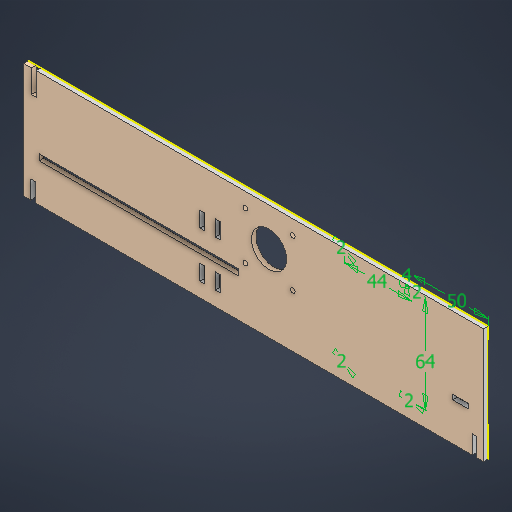
# Autodesk Inventor part: Sideboard
Saved by Autodesk Inventor 2027 (Build 310192000, 192)
## iProperties
Created: 2026-05-09
Part Number: Sideboard
Material: Generic
Document SubType Name: Modeling
Designer: alexy
Density: 1 g/cm^3
Appearance: Default
Author: alexy
Autodesk Inventor part; units mm, degrees
ref_plane "YZ Plane" through (0, 0, 0) normal (1, 0, 0) x (0, 1, 0)
ref_plane "XZ Plane" through (0, 0, 0) normal (0, 1, 0) x (-1, 0, 0)
ref_plane "XY Plane" through (0, 0, 0) normal (0, 0, 1) x (1, 0, 0)
sketch "Sketch1" plane through (0, 0, 0) normal (0, 0, 1) x (1, 0, 0)
  line L0 (0, 0) -> (300, 0)
  line L1 (300, 0) -> (300, 65)
  line L2 (300, 65) -> (0, 65)
  line L3 (0, 65) -> (0, 0)
  circle A0 centre (144.5, 55.5) radius 1.55
  circle A1 centre (144.5, 24.5) radius 1.55
  circle A2 centre (175.5, 55.5) radius 1.55
  circle A3 centre (175.5, 24.5) radius 1.55
  circle A4 centre (160, 40) radius 11.5
  line L4 (10, 19) -> (140, 19)
  line L5 (140, 19) -> (140, 15)
  line L6 (140, 15) -> (10, 15)
  line L7 (10, 15) -> (10, 19)
  line L8 (0, 65) -> (39.6145, 65)
  line L9 (8.1, 50) -> (5, 50)
  line L10 (5, 50) -> (5, 65)
  line L11 (5, 65) -> (8.1, 65)
  line L12 (8.1, 65) -> (8.1, 50)
  line L13 (8.1, 50) -> (5, 65) construction
  line L14 (5, 50) -> (8.1, 65) construction
  line L15 (0, 65) -> (50, 65)
  line L16 (0, 0) -> (0, -10)
  line L17 (0, -10) -> (300, -10)
  line L18 (300, -10) -> (300, 0)
  point P0 (6.55, 57.5)
  point P1 (5, 57.5)
  point P2 (8.1, 57.5)
  point P3 (10, 17)
  point P4 (140, 17)
  dimension "d1" = 3.1
  dimension "d2" = 3.1
  dimension "d3" = 3.1
  dimension "d4" = 3.1
  dimension "d5" = 31
  dimension "d7" = 23
  dimension "d8" = 15.5
  dimension "d9" = 15.5
  dimension "d10" = 65
  dimension "d11" = 31
  dimension "d13" = 40
  dimension "d54" = 300
  dimension "d55" = 3.1
  dimension "d56" = 5
  dimension "d59" = 130
  dimension "d93" = 15
  dimension "d106" = 20
  dimension "d107" = 10
  dimension "d201" = 4
  dimension "d202" = 10
  dimension "d274" = 15
  constraints: 38 end point, 6 midpoint, 6 parallel, 5 centre point, 5 perpendicular, 4 horizontal, 3 horizontal alignment, 2 vertical alignment, 1 vertical
  measures "d1" diameter of A0
  measures "d2" diameter of A1
  measures "d3" diameter of A2
  measures "d4" diameter of A3
  measures "d5" distance of A1.centre A3.centre
  measures "d7" diameter of A4
  measures "d8" horizontal distance of A0.centre A4.centre
  measures "d9" horizontal distance of A4.centre A3.centre
  measures "d10" distance of L0.end L1.end
  measures "d11" distance of A3.centre A2.centre
  measures "d13" distance from line of L0 A4.centre
  measures "d54" distance of L0.end L0.start
  measures "d55" distance of L10.end L11.end
  measures "d56" distance between parallel lines of L3 L10
  measures "d59" distance of L5.end L6.end
  measures "d93" distance between parallel lines of L0 L6
  measures "d106" horizontal distance of point (140, 17) A4.centre
  measures "d107" distance from line of L3 point (10, 17)
  measures "d201" distance of L6.end L4.start
  measures "d202" distance of L0.start L16.end
  measures "d274" distance from line of L15 L9.start
extrude "Extrusion1" add sketch "Sketch1" along normal blind 3 contours L3 L2 L10 L9 L12 L1 L0 | L0 L18 L17 L16
sketch "Sketch7" plane through (0, 0, 3) normal (0, 0, 1) x (1, 0, 0)
  line L0 (300, 65) -> (0, 65) projected
  circle A0 centre (144.5, 55.5) radius 1.55 projected
  line L1 (124.95, 39.55) -> (128.05, 39.55)
  line L2 (128.05, 39.55) -> (128.05, 29.45)
  line L3 (128.05, 29.45) -> (124.95, 29.45)
  line L4 (124.95, 29.45) -> (124.95, 39.55)
  line L5 (124.95, 39.55) -> (128.05, 29.45) construction
  line L6 (128.05, 39.55) -> (124.95, 29.45) construction
  line L7 (114.95, 39.55) -> (118.05, 39.55)
  line L8 (118.05, 39.55) -> (118.05, 29.45)
  line L9 (118.05, 29.45) -> (114.95, 29.45)
  line L10 (114.95, 29.45) -> (114.95, 39.55)
  line L11 (114.95, 39.55) -> (118.05, 29.45) construction
  line L12 (118.05, 39.55) -> (114.95, 29.45) construction
  line L13 (128.1, 9.55) -> (128.1, -0.55)
  line L14 (128.1, -0.55) -> (124.9, -0.55)
  line L15 (124.9, 9.55) -> (128.1, 9.55)
  line L16 (124.9, -0.55) -> (124.9, 9.55)
  line L17 (124.9, 9.55) -> (128.1, -0.55) construction
  line L18 (128.1, 9.55) -> (124.9, -0.55) construction
  line L19 (118.1, 9.55) -> (118.1, -0.55)
  line L20 (118.1, -0.55) -> (114.9, -0.55)
  line L21 (114.9, 9.55) -> (118.1, 9.55)
  line L22 (114.9, -0.55) -> (114.9, 9.55)
  line L23 (114.9, 9.55) -> (118.1, -0.55) construction
  line L24 (118.1, 9.55) -> (114.9, -0.55) construction
  line L25 (0, -10) -> (300, -10) projected
  line L26 (300, -10) -> (300, 65) projected
  circle A1 centre (144.5, 24.5) radius 1.55 projected
  point P0 (0, 0)
  point P1 (242, 62)
  point P2 (126.5, 34.5)
  point P3 (116.5, 34.5)
  point P4 (126.5, 4.5)
  point P5 (116.5, 4.5)
  point P6 (114.9, 4.5)
  point P7 (150, -10)
  dimension "d155" = 10.1
  dimension "d183" = 3.2
  dimension "d185" = 3.2
  dimension "d192" = 10
  dimension "d267" = 10.1
  dimension "d268" = 18
  dimension "d269" = 10
  dimension "d270" = 3.1
  dimension "d271" = 3.1
  dimension "d272" = 10
  dimension "d273" = 30
  constraints: 48 end point, 10 midpoint, 8 parallel, 4 horizontal, 4 horizontal alignment, 4 perpendicular, 1 vertical alignment, 1 other
  measures "d155" distance of L4.start L1.start
  measures "d183" distance of L13.end L16.start
  measures "d185" distance of L19.end L24.end
  measures "d192" distance of point (126.5, 4.5) point (116.5, 4.5)
  measures "d267" distance of L18.start L13.end
  measures "d268" horizontal distance of point (126.5, 34.5) A1.centre
  measures "d269" vertical distance of A1.centre point (126.5, 34.5)
  measures "d270" distance of L1.start L1.end
  measures "d271" distance of L7.start L7.end
  measures "d272" distance of point (116.5, 34.5) point (126.5, 34.5)
  measures "d273" distance of point (116.5, 4.5) point (116.5, 34.5)
extrude "Extrusion6" cut sketch "Sketch7" against normal blind 3 contours L1 L2 L3 L4 | L7 L8 L9 L10 | L13 L14 L16 L15 | L19 L20 L22 L21
sketch "Sketch8" plane through (0, 0, 3) normal (0, 0, 1) x (1, 0, 0)
  line L0 (0, -10) -> (300, -10) projected
  line L1 (279.8, 18) -> (290, 18)
  line L2 (290, 18) -> (290, 14.8)
  line L3 (290, 14.8) -> (279.8, 14.8)
  line L4 (279.8, 14.8) -> (279.8, 18)
  line L5 (300, -10) -> (300, 65) projected
  line L6 (4.5, 2) -> (7.5, 2)
  line L7 (7.5, 2) -> (7.5, -10)
  line L8 (7.5, -10) -> (4.5, -10)
  line L9 (4.5, -10) -> (4.5, 2)
  line L10 (4.5, 2) -> (7.5, -10) construction
  line L11 (7.5, 2) -> (4.5, -10) construction
  line L12 (295.5, 2) -> (292.5, 2)
  line L13 (292.5, 2) -> (292.5, -10)
  line L14 (292.5, -10) -> (295.5, -10)
  line L15 (295.5, -10) -> (295.5, 2)
  line L16 (295.5, 2) -> (292.5, -10) construction
  line L17 (292.5, 2) -> (295.5, -10) construction
  point P0 (0, 0)
  point P1 (6, -4)
  point P2 (4.5, -4)
  point P3 (294, -4)
  dimension "d219" = 28
  dimension "d220" = 3.2
  dimension "d221" = 10.2
  dimension "d222" = 10
  dimension "d223" = 3
  dimension "d247" = 3
  dimension "d248" = 6
  dimension "d249" = 12
  dimension "d263" = 6
  constraints: 32 end point, 6 parallel, 5 midpoint, 3 horizontal, 3 perpendicular, 2 horizontal alignment, 1 point on line
  measures "d219" distance between parallel lines of L0 L1
  measures "d220" distance of L3.end L1.start
  measures "d221" distance of L2.end L3.end
  measures "d222" distance between parallel lines of L5 L2
  measures "d223" distance of L7.end L8.end
  measures "d247" distance between parallel lines of L13 L15
  measures "d248" distance from line of L5 point (294, -4)
  measures "d249" distance of L14.end L12.start
  measures "d263" horizontal distance of L0.start point (6, -4)
extrude "Extrusion7" cut sketch "Sketch8" against normal blind 3
sketch "Sketch10" plane through (0, 0, 0) normal (0, 0, -1) x (-1, 0, 0)
  circle A0 centre (-250, 61) radius 1
  circle A1 centre (-206, 61) radius 1
  circle A2 centre (-206, -3) radius 1
  circle A3 centre (-250, -3) radius 1
  line L0 (-300, 65) -> (0, 65) projected
  line L1 (-300, -10) -> (-300, 65) projected
  point P0 (0, 0)
  dimension "d255" = 2
  dimension "d256" = 4
  dimension "d257" = 50
  dimension "d258" = 2
  dimension "d259" = 2
  dimension "d260" = 2
  dimension "d261" = 64
  dimension "d262" = 44
  constraints: 4 centre point, 2 horizontal alignment, 2 vertical alignment
  measures "d255" diameter of A0
  measures "d256" distance from line of L0 A0.centre
  measures "d257" distance from line of L1 A0.centre
  measures "d258" diameter of A1
  measures "d259" diameter of A2
  measures "d260" diameter of A3
  measures "d261" distance of A3.centre A0.centre
  measures "d262" distance of A0.centre A1.centre
body "Solid1"
